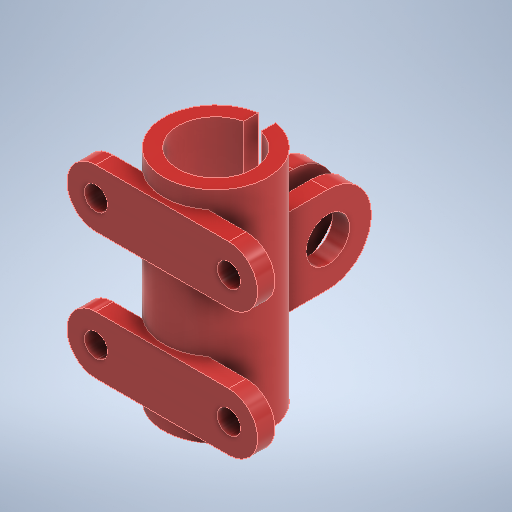
# Autodesk Inventor part: cad@68
Saved by Autodesk Inventor 2025.2 (Build 292293000, 293)
## iProperties
Created: 2025-04-22
Part Number: cad@68
Material: Generic
Document SubType Name: Modeling
Designer: spars
Density: 1 g/cm^3
Appearance: Orange-Red
Author: spars
Autodesk Inventor part; units mm, degrees
ref_plane "YZ Plane" through (0, 0, 0) normal (1, 0, 0) x (0, 1, 0)
sketch "Sketch1" plane through (0, 0, 0) normal (0, 0, 1) x (1, 0, 0)
  line L0 (-57.5, -7.2529) -> (57.5, -7.2529) construction
  line L1 (-57.5, -32.2529) -> (57.5, -32.2529)
  line L2 (57.5, 17.7471) -> (-57.5, 17.7471)
  arc A0 (-57.5, 17.7471) -> (-57.5, -32.2529) centre (-57.5, -7.2529) ccw
  arc A1 (57.5, -32.2529) -> (57.5, 17.7471) centre (57.5, -7.2529) ccw
  circle A2 centre (-57.5, -7.2529) radius 10
  circle A3 centre (57.5, -7.2529) radius 10
  line L3 (-57.5, -117.2529) -> (57.5, -117.2529) construction
  line L4 (-57.5, -142.2529) -> (57.5, -142.2529)
  line L5 (57.5, -92.2529) -> (-57.5, -92.2529)
  arc A4 (-57.5, -92.2529) -> (-57.5, -142.2529) centre (-57.5, -117.2529) ccw
  arc A5 (57.5, -142.2529) -> (57.5, -92.2529) centre (57.5, -117.2529) ccw
  circle A6 centre (-57.5, -117.2529) radius 10
  circle A7 centre (57.5, -117.2529) radius 10
  point P0 (0, 0)
  point P1 (0, -7.2529)
  point P2 (0, -117.2529)
  point P3 (82.5, -117.2529)
  point P4 (-82.5, -117.2529)
  dimension "d0" = 115
  dimension "d1" = 25
  dimension "d2" = 20
  dimension "d3" = 20
  dimension "d4" = 115
  dimension "d5" = 25
  dimension "d6" = 20
  dimension "d7" = 20
  dimension "d8" = 110
  dimension "d11" = 165
  constraints: 16 end point, 10 point on circle, 8 centre point, 8 tangent, 4 coincident, 2 horizontal, 2 midpoint, 2 parallel
  measures "d0" distance of L0.end L0.start
  measures "d1" radius of A0
  measures "d2" diameter of A2
  measures "d3" diameter of A3
  measures "d4" distance of L3.end L3.start
  measures "d5" radius of A4
  measures "d6" diameter of A6
  measures "d7" diameter of A7
  measures "d8" distance of A6.centre A2.centre
  measures "d11" distance of point (82.5, -117.253) point (-82.5, -117.253)
extrude "Extrusion1" add sketch "Sketch1" along normal blind 15
sketch "Sketch2" plane through (0, 0, 0) normal (0, 0, -1) x (-1, 0, 0)
  point P0 (0, 0)
sketch "Sketch3" plane through (0, 0, 0) normal (0, 0, -1) x (-1, 0, 0)
  point P0 (0, 0)
sketch "Sketch4" plane through (-57.5, 17.7471, 0) normal (0, 1, 0) x (1, 0, 0)
  arc A0 (46.2455, 79.3706) -> (61.2455, 79.3706) centre (53.7455, 35) ccw
  line L0 (115, 0) -> (0, 0) projected
  arc A1 (46.2455, 66.6228) -> (61.2455, 66.6228) centre (53.7455, 35) ccw
  line L1 (46.2455, -10) -> (61.2455, 80) construction
  line L2 (61.2455, -10) -> (46.2455, 80) construction
  line L3 (46.2455, 79.3706) -> (46.2455, 66.6228)
  line L4 (61.2455, 66.6228) -> (61.2455, 79.3706)
  point P0 (57.5, 0)
  dimension "d12" = 90
  dimension "d13" = 35
  dimension "d14" = 65
  dimension "d15" = 15
  dimension "d16" = 90
  constraints: 8 end point, 4 point on circle, 2 centre point, 2 midpoint, 1 coincident, 1 parallel
  measures "d12" diameter of A0
  measures "d13" distance from line of L0 A0.centre
  measures "d14" diameter of A1
  measures "d15" distance of L2.end L1.end
  measures "d16" distance of L1.end L2.start
extrude "Extrusion2" add sketch "Sketch4" along normal blind 15 and the other way blind 175
sketch "Sketch5" plane through (0, 0, 0) normal (1, 0, 0) x (0, 1, 0)
  point P0 (0, 0)
ref_plane "Work Plane1" through (3.7455, 17.7471, -79.3706) normal (1, 0, 0) x (0, 1, 0)
sketch "Sketch6" plane through (3.7455, 17.7471, -79.3706) normal (1, 0, 0) x (0, 1, 0)
  circle A0 centre (-80, -30.1908) radius 18.75
  arc A1 (-117.5, -30.1908) -> (-42.5, -30.1908) centre (-80, -30.1908) ccw
  line L0 (-117.5, -30.1908) -> (-117.5, 12.3826)
  line L1 (-117.5, 12.3826) -> (-42.5, 12.3826)
  line L2 (-42.5, 12.3826) -> (-42.5, -30.1908)
  point P0 (-17.7471, 79.3706)
  dimension "d21" = 37.5
  dimension "d22" = 75
  constraints: 6 end point, 2 centre point, 2 perpendicular, 2 point on circle, 1 coincident, 1 tangent, 1 vertical
  measures "d21" diameter of A0
  measures "d22" diameter of A1
extrude "Extrusion3" add sketch "Sketch6" along normal blind 15
ref_plane "Work Plane2" through (-3.7545, -157.2529, -79.3706) normal (1, 0, 0) x (0, 0, -1)
mirror "Mirror1" about plane through (-3.7545, -157.2529, -79.3706) normal (1, 0, 0) of "Extrusion3"
body "Solid1"
